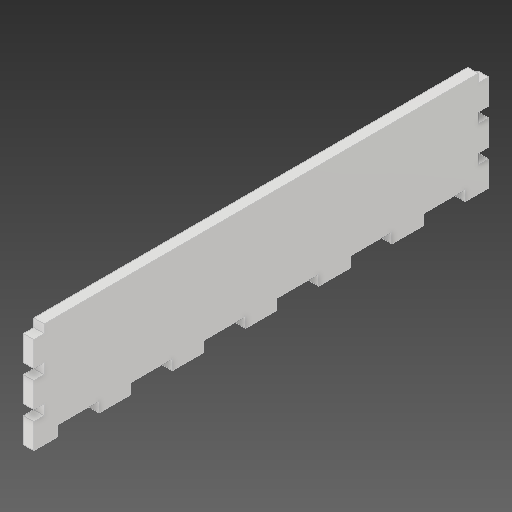
# Autodesk Inventor part: Front_Back
Saved by Autodesk Inventor 2018 (Build 220112000, 112)
## iProperties
Created: 2018-03-12
Part Number: Front_Back
Material: UHMW, White
Document SubType Name: Modeling
Designer: gaine
Density: 0.94 g/cm^3
Appearance: Smooth - White
Author: gaine
Autodesk Inventor part; units mm, degrees
ref_plane "YZ Plane" through (0, 0, 0) normal (1, 0, 0) x (0, 1, 0)
ref_plane "XZ Plane" through (0, 0, 0) normal (0, 1, 0) x (-1, 0, 0)
ref_plane "XY Plane" through (0, 0, 0) normal (0, 0, 1) x (1, 0, 0)
sketch "Sketch1" plane through (0, 0, 0) normal (1, 0, 0) x (0, 1, 0)
  line L0 (44.6473, -162.2528) -> (44.6473, 101.2722)
  line L1 (-18.8527, 107.6222) -> (-3.6127, 107.6222)
  line L2 (-3.6127, 107.6222) -> (-3.6127, 101.2722)
  line L3 (-18.8527, 101.0377) -> (-18.8527, 107.6222)
  line L4 (2.7373, 107.6222) -> (17.9773, 107.6222)
  line L5 (17.9773, 107.6222) -> (17.9773, 101.2722)
  line L6 (2.7373, 101.2722) -> (2.7373, 107.6222)
  line L7 (24.3273, 107.6222) -> (39.5673, 107.6222)
  line L8 (39.5673, 107.6222) -> (39.5673, 101.2722)
  line L9 (24.3273, 101.2722) -> (24.3273, 107.6222)
  line L10 (39.5673, 101.2722) -> (44.6473, 101.2722)
  line L11 (24.3273, 101.2722) -> (17.9773, 101.2722)
  line L12 (2.7373, 101.2722) -> (-3.6127, 101.2722)
  line L13 (44.6473, -30.4903) -> (-18.8527, -30.4903) construction
  line L14 (-3.6127, -168.6028) -> (-3.6127, -162.2528)
  line L15 (17.9773, -168.6028) -> (17.9773, -162.2528)
  line L16 (2.7373, -162.2528) -> (2.7373, -168.6028)
  line L17 (39.5673, -168.6028) -> (39.5673, -162.2528)
  line L18 (24.3273, -162.2528) -> (24.3273, -168.6028)
  line L19 (39.5673, -162.2528) -> (44.6473, -162.2528)
  line L20 (24.3273, -162.2528) -> (17.9773, -162.2528)
  line L21 (2.7373, -162.2528) -> (-3.6127, -162.2528)
  line L22 (24.3273, -168.6028) -> (39.5673, -168.6028)
  line L23 (-18.8527, -168.6028) -> (-3.6127, -168.6028)
  line L24 (2.7373, -168.6028) -> (17.9773, -168.6028)
  line L25 (-3.6127, 107.6222) -> (-18.8527, 107.6222)
  line L26 (39.5673, 107.6222) -> (24.3273, 107.6222)
  line L27 (17.9773, 107.6222) -> (2.7373, 107.6222)
  line L28 (-18.8527, -20.9653) -> (-12.5027, -20.9653)
  line L29 (-12.5027, -20.9653) -> (-12.5027, 4.4347)
  line L30 (-12.5027, 4.4347) -> (-18.8527, 4.4347)
  line L31 (-18.8527, 23.4847) -> (-12.5027, 23.4847)
  line L32 (-12.5027, 23.4847) -> (-12.5027, 48.8847)
  line L33 (-12.5027, 48.8847) -> (-18.8527, 48.8847)
  line L34 (-18.8527, 67.9347) -> (-12.5027, 67.9347)
  line L35 (-12.5027, 67.9347) -> (-12.5027, 93.3347)
  line L36 (-12.5027, 93.3347) -> (-18.8527, 93.3347)
  line L37 (-3.6127, -168.6028) -> (-3.6127, -162.2528)
  line L38 (2.7373, -162.2528) -> (-3.6127, -162.2528)
  line L39 (-18.8527, -40.0153) -> (-12.5027, -40.0153)
  line L40 (-12.5027, -40.0153) -> (-12.5027, -65.4153)
  line L41 (-12.5027, -65.4153) -> (-18.8527, -65.4153)
  line L42 (-18.8527, -84.4653) -> (-12.5027, -84.4653)
  line L43 (-12.5027, -84.4653) -> (-12.5027, -109.8653)
  line L44 (-12.5027, -109.8653) -> (-18.8527, -109.8653)
  line L45 (-18.8527, -128.9153) -> (-12.5027, -128.9153)
  line L46 (-12.5027, -128.9153) -> (-12.5027, -154.3153)
  line L47 (-12.5027, -154.3153) -> (-18.8527, -154.3153)
  line L48 (-18.8527, 107.6222) -> (-18.8527, 93.3347)
  line L49 (-18.8527, 67.9347) -> (-18.8527, 48.8847)
  line L50 (-18.8527, 23.4847) -> (-18.8527, 4.4347)
  line L51 (-18.8527, -20.9653) -> (-18.8527, -40.0153)
  line L52 (-18.8527, -65.4153) -> (-18.8527, -84.4653)
  line L53 (-18.8527, -109.8653) -> (-18.8527, -128.9153)
  line L54 (-18.8527, -154.3153) -> (-18.8527, -168.6028)
  point P0 (0, 0)
  dimension "d2" = 15.24
  dimension "d3" = 6.35
  dimension "d4" = 15.24
  dimension "d5" = 6.35
  dimension "d7" = 15.24
  dimension "d8" = 9.525
  dimension "d9" = 19.05
  dimension "d10" = 19.05
  dimension "d12" = 25.4
  dimension "d13" = 25.4
  dimension "d14" = 25.4
  dimension "d16" = 6.35
  dimension "d17" = 6.35
  dimension "d20" = 276.225
  constraints: 110 end point, 27 perpendicular, 23 symmetric about line, 22 parallel, 11 horizontal, 6 collinear, 4 point on line, 2 midpoint
  measures "d2" distance between parallel lines of L3 L2
  measures "d3" distance between parallel lines of L2 L6
  measures "d4" distance between parallel lines of L6 L5
  measures "d5" distance between parallel lines of L5 L9
  measures "d7" distance between parallel lines of L8 L9
  measures "d8" distance between parallel lines of L13 L28
  measures "d9" distance between parallel lines of L31 L30
  measures "d10" distance between parallel lines of L34 L33
  measures "d12" distance between parallel lines of L30 L28
  measures "d13" distance between parallel lines of L33 L31
  measures "d14" distance between parallel lines of L36 L34
  measures "d16" distance between parallel lines of L12 L1
  measures "d17" distance between parallel lines of L48 L35
  measures "d20" distance between parallel lines of L22 L7
extrude "Extrusion1" add sketch "Sketch1" along normal blind 6.35
equation "\"d10\" = d9"
equation "\"d13\" = d12"
equation "\"d14\" = d12"
body "Solid1"
